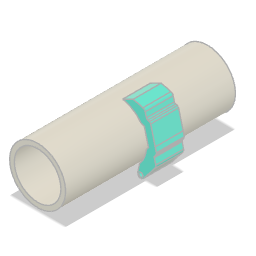
Payload Clamp Prototype (Autodesk Fusion 360 design; units mm, degrees)
Autodesk Fusion 360 part; units mm, degrees
sketch "Sketch1" plane through (0, 0, 0) normal (0, 0, 1) x (1, 0, 0)
  circle A0 centre (0, 50) radius 30
  circle A1 centre (0, 50) radius 25
  dimension "d1" = 60
  dimension "d2" = -5
  measures "d1" diameter of A0
extrude "Extrude1" add sketch "Sketch1" along normal blind 175 makes body 1
extrude "Extrude2" add sketch "Sketch1" against normal blind 7.5 contours A0 | A1 bodies 1
sketch "Sketch2" plane through (0, 0, -7.5) normal (0, 0, -1) x (-1, 0, 0)
  circle A0 centre (0, 50) radius 30
  circle A1 centre (0, 50) radius 30
  line L0 (0, 20) -> (0, 25)
  line L1 (-18.3303, 25) -> (-16.5831, 25)
  line L2 (-23.608, 29.9087) -> (-34.5881, 29.9087)
  line L3 (-30.7813, 46.3244) -> (-39.3496, 42.8163)
  circle A2 centre (0, 50) radius 31
  line L4 (-24.7175, 68.7094) -> (-27.8021, 78.7583)
  line L5 (-5.2295, 80.5557) -> (-16.7866, 86.3071)
  arc A3 (-16.7866, 86.3071) -> (-27.8021, 78.7583) centre (0, 50) ccw
  arc A4 (-39.3496, 42.8163) -> (-34.5881, 29.9087) centre (0, 50) ccw
  line L6 (5.2295, 80.5557) -> (16.7866, 86.3071)
  arc A5 (27.8021, 78.7583) -> (16.7866, 86.3071) centre (0, 50) ccw
  line L7 (24.7175, 68.7094) -> (27.8021, 78.7583)
  line L8 (30.7813, 46.3244) -> (39.3496, 42.8163)
  arc A6 (34.5881, 29.9087) -> (39.3496, 42.8163) centre (0, 50) ccw
  line L9 (23.608, 29.9087) -> (34.5881, 29.9087)
  dimension "d8" = 1
  constraint coincident A0 L0.start
  constraint concentric A0 A3
  constraint coincident L2.end A3
  constraint horizontal L2
  constraint coincident L3.end A3
  constraint coincident A2 L3.start
  constraint coincident A2 L2.start
  constraint coincident A2 L4.start
  constraint coincident A2 L5.start
  constraint concentric A3 A4
  constraint coincident A0 L1.end
  constraint coincident A2 L1.start
  constraint symmetric L0 L2.end A6.start
  constraint symmetric L0 L3.end L8.end
  constraint symmetric L0 L3.start L8.start
  constraint symmetric L0 L2.start L9.start
  constraint symmetric L0 L4.start L7.start
  constraint symmetric L0 L4.end A5.start
  constraint symmetric L0 L5.start L6.start
  constraint symmetric L0 L5.end L6.end
  constraint symmetric L0 A3 A5
  constraint symmetric L0 A4 A6
extrude "Extrude3" add sketch "Sketch2" against normal blind 30 separate body contours L2 L3 A2 A4 | A2 L4 L5 A3 | A2 L8 A6 L9 | A2 L6 A5 L7 makes body 2 at (-7.7659, 80.0115, 12.5) makes body 3 at (30.5651, 44.8256, 2.5) makes body 4 at (23.9131, 69.7273, 12.5) makes body 5 at (-29.4818, 40.4174, 12.5)
sketch "Sketch3" plane through (0, 0, -7.5) normal (0, 0, -1) x (-1, 0, 0)
  line L0 (-5.2295, 80.5557) -> (-16.7866, 86.3071)
  arc A0 (-16.7866, 86.3071) -> (-27.8021, 78.7583) centre (0, 50) ccw
  line L1 (-27.8021, 78.7583) -> (-24.7175, 68.7094)
  arc A1 (-5.2295, 80.5557) -> (-24.7175, 68.7094) centre (0, 50) ccw
  line L2 (-30.7813, 46.3244) -> (-39.3496, 42.8163)
  arc A2 (-39.3496, 42.8163) -> (-34.5881, 29.9087) centre (0, 50) ccw
  line L3 (-34.5881, 29.9087) -> (-23.608, 29.9087)
  arc A3 (-30.7813, 46.3244) -> (-23.608, 29.9087) centre (0, 50) ccw
  circle A4 centre (0, 50) radius 30
  circle A5 centre (-37.528, 36.1563) radius 2.5
  arc A6 (-40.9187, 37.0242) -> (-39.5025, 33.2664) centre (-37.528, 36.1563) ccw
  circle A7 centre (-26.2598, 80.1732) radius 2.5
  arc A8 (-27.1572, 83.5562) -> (-29.6505, 81.0412) centre (-26.2598, 80.1732) ccw
  line L4 (-40.9187, 37.0242) -> (-29.6505, 81.0412)
  line L5 (-31.0003, 57.936) -> (-28.6395, 67.1583)
  line L6 (-31.0003, 57.936) -> (-33.1425, 49.5681)
  line L7 (-27.1572, 83.5562) -> (-16.7866, 86.3071)
  line L8 (-39.5025, 33.2664) -> (-34.5881, 29.9087)
  line L9 (-25.7516, 72.078) -> (-24.7175, 68.7094)
  line L10 (-33.1425, 49.5681) -> (-30.7813, 46.3244)
  line L11 (-24.7175, 68.7094) -> (-28.6395, 67.1583)
  dimension "d11" = 5
  dimension "d12" = 7
  dimension "d13" = 5
  dimension "d14" = 7
  constraint midpoint A2 A5.centre
  constraint concentric A5 A6
  constraint coincident A0 A7.centre
  constraint concentric A7 A8
  constraint tangent A6 L4
  constraint coincident A8 L4.end
  constraint tangent A8 L4
  constraint tangent A8 L7
  constraint coincident L0.end A0.start
  constraint tangent A6 L8
  constraint coincident A2.end L3.start
  constraint coincident L4 A8.end
  constraint coincident L1 L9.start
  constraint coincident L1.end A1.end
  constraint coincident L2.start A3.start
  measures "d11" diameter of A5
  measures "d12" diameter of A6
  measures "d13" diameter of A7
  measures "d14" diameter of A8
extrude "Extrude4" add sketch "Sketch3" against normal blind 30 contours A0 L1 L2 A2 A5 A6 A7 A8 L4 L5 L6 L7 L8 L9 L10 L11 bodies 3 4
extrude "Extrude5" cut sketch "Sketch3" against normal blind 30 contours A0 L1 A7 | A2 A5 picked at (-25.5221, 79.7151) picked at (-36.7243, 36.3975) bodies 3
delete_body "RemoveBody1" bodies 5
delete_body "RemoveBody2" bodies 2
copy_body "CopyPasteBodies1" bodies 3 makes body 6
move_body "Move1" bodies 6 to x (0.707107, -0.707107, 0) y (0.707107, 0.707107, 0) z (0, 0, 1) at (-7.5036, 30.0552, 0)
sketch "Sketch4" plane through (0, 0, -7.5) normal (0, 0, -1) x (-1, 0, 0)
  circle A0 centre (0, 50) radius 30
  circle A1 centre (-37.528, 36.1563) radius 2.5
  circle A2 centre (-44.5991, 29.0852) radius 2.5
  circle A3 centre (-24.8785, 20.0964) radius 2.5
  line L0 (-34.7785, 38.3219) -> (-22.1289, 22.2621)
  line L1 (-40.2775, 33.9906) -> (-27.628, 17.9307)
  arc A4 (-34.7785, 38.3219) -> (-40.2775, 33.9906) centre (-37.528, 36.1563) ccw
  arc A5 (-27.628, 17.9307) -> (-22.1289, 22.2621) centre (-24.8785, 20.0964) ccw
  dimension "d20" = 5
  dimension "d21" = 7
  dimension "d22" = 7
  constraint concentric A3 A5
  constraint concentric A1 A4
  constraint tangent L0 A4
  constraint tangent L0 A5
  constraint tangent L1 A4
  constraint tangent L1 A5
  constraint parallel L0 L1
  measures "d20" diameter of A3
  measures "d21" diameter of A5
  measures "d22" diameter of A4
extrude "Extrude6" add sketch "Sketch4" along normal blind 7.5 separate body contours L0 L1 A4 A5 makes body 7
move_body "Move2" bodies 7 to x (0.906308, -0.422618, 0) y (0.422618, 0.906308, 0) z (0, 0, 1) at (-6.1622, 12.397, 0)
move_body "Move3" bodies 6 to x (1, 0, 0) y (0, 1, 0) z (0, 0, 1) at (-1.5, 0.25, 0)
move_body "Move4" bodies 7 to x (0.906308, 0.422618, 0) y (-0.422618, 0.906308, 0) z (0, 0, 1) at (10.824, -8.6312, 0)
sketch "Sketch5" plane through (0, 0, -7.5) normal (0, 0, -1) x (-1, 0, 0)
  circle A0 centre (-26.2598, 80.1732) radius 2.5
  line L0 (-34.5881, 29.9087) -> (-23.608, 29.9087)
  arc A1 (-30.7813, 46.3244) -> (-23.608, 29.9087) centre (0, 50) ccw
  line L1 (-30.7813, 46.3244) -> (-33.1425, 49.5681)
  line L2 (-33.1425, 49.5681) -> (-28.6395, 67.1583)
  line L3 (-28.6395, 67.1583) -> (-24.7175, 68.7094)
  arc A2 (-5.2295, 80.5557) -> (-24.7175, 68.7094) centre (0, 50) ccw
  line L4 (-5.2295, 80.5557) -> (-16.7866, 86.3071)
  line L5 (-16.7866, 86.3071) -> (-27.1572, 83.5562)
  arc A3 (-27.1572, 83.5562) -> (-29.6505, 81.0412) centre (-26.2598, 80.1732) ccw
  line L6 (-29.6505, 81.0412) -> (-40.9187, 37.0242)
  arc A4 (-40.9187, 37.0242) -> (-39.5025, 33.2664) centre (-37.528, 36.1563) ccw
  line L7 (-39.5025, 33.2664) -> (-34.5881, 29.9087)
  circle A5 centre (-37.528, 36.1563) radius 2.5
  circle A6 centre (-26.2598, 80.1732) radius 2.5
  line L8 (-58.0759, 36.6699) -> (-29.6505, 81.0412)
  line L9 (-23.3075, 78.2934) -> (-49.9806, 36.4014)
  circle A7 centre (-24.8785, 20.0964) radius 2.5
  line L10 (-56.5521, 31.863) -> (-26.4306, 16.9594)
  line L11 (-23.3282, 23.2344) -> (-49.9806, 36.4014)
  arc A8 (-23.3075, 78.2934) -> (-29.6505, 81.0412) centre (-26.2598, 80.1732) ccw
  arc A9 (-26.4306, 16.9594) -> (-23.3282, 23.2344) centre (-24.8785, 20.0964) ccw
  arc A10 (-57.8029, 37.0962) -> (-56.5521, 31.863) centre (-55, 35) ccw
  dimension "d25" = 7
  dimension "d26" = 7
  dimension "d27" = 7
  constraint concentric A6 A8
  constraint coincident L8.start A10
  constraint coincident A3.end L6.start
  constraint tangent L9 A8
  constraint concentric A7 A9
  constraint tangent L10 A10
  constraint tangent L10 A9
  constraint tangent L11 A9
  constraint coincident L8 A10.start
  measures "d25" diameter of A8
  measures "d26" diameter of A10
  measures "d27" diameter of A9
extrude "Extrude7" add sketch "Sketch5" along normal blind 7.5 separate body contours L6 L8 L9 L10 L11 A9 A10 | A3 L6 L9 A8 makes body 8
delete_body "RemoveBody3" bodies 8
move_body "Move5" bodies 7 to x (1, 0, 0) y (0, 1, 0) z (0, 0, 1) at (0, 0, 38)
extrude "Extrude8" add 1 faces at (35.3299, 28.5468, 30.5) along direction (0, 0, 1) blind 20 on bodies 7 bodies 7
sketch "Sketch6" plane through (0, 0, 23) normal (0, 0, -1) x (-1, 0, 0)
  circle A0 centre (-37.528, 36.1563) radius 2.5
  circle A1 centre (-24.8785, 20.0964) radius 2.5
  arc A2 (-34.7785, 38.3219) -> (-40.2775, 33.9906) centre (-37.528, 36.1563) ccw
  line L0 (-40.2775, 33.9906) -> (-27.628, 17.9307)
  arc A3 (-27.628, 17.9307) -> (-22.1289, 22.2621) centre (-24.8785, 20.0964) ccw
  line L1 (-22.1289, 22.2621) -> (-34.7785, 38.3219)
  circle A4 centre (-24.8785, 20.0964) radius 2.5
  line L2 (-21.4618, 15.0964) -> (-14.8785, 15.0964)
  line L3 (-14.8785, 15.0964) -> (-14.8785, 10.0964)
  line L4 (-14.8785, 10.0964) -> (-24.8785, 10.0964)
  line L5 (-28.3785, 15.0964) -> (-34.8785, 15.0964)
  line L6 (-34.8785, 15.0964) -> (-34.8785, 10.0964)
  line L7 (-34.8785, 10.0964) -> (-24.8785, 10.0964)
  line L8 (-21.3789, 20.0377) -> (-21.4618, 15.0964)
  line L9 (-28.3785, 20.0964) -> (-28.3785, 15.0964)
  arc A5 (-21.3789, 20.0377) -> (-28.3785, 20.0964) centre (-24.8785, 20.0964) ccw
  dimension "d32" = 7
  constraint concentric A4 A5
  constraint horizontal L2
  constraint vertical L3
  constraint horizontal L4
  constraint horizontal L5
  constraint vertical L6
  constraint horizontal L7
  constraint coincident A3 L8.start
  constraint tangent L8 A5
  constraint tangent L9 A5
  constraint perpendicular L5 L9
  measures "d32" diameter of A5
extrude "Extrude9" add sketch "Sketch6" along normal blind 8 separate body contours L0 A3 L9 A5 | L0 A3 L2 L3 L4 L5 L6 L7 L8 L9 makes body 9
fillet "Fillet1" radius 4 2 edges at (28.3785, 15.0964, 19) (21.4618, 15.0964, 19) on bodies 9
sketch "Sketch7" plane through (0, 0, 23) normal (0, 0, 1) x (1, 0, 0)
  circle A0 centre (24.8785, 20.0964) radius 2.5
  line L0 (21.3789, 20.0377) -> (21.3936, 19.1635)
  arc A1 (17.3942, 15.0964) -> (21.3936, 19.1635) centre (17.3942, 19.0964) ccw
  line L1 (17.3942, 15.0964) -> (14.8785, 15.0964)
  line L2 (14.8785, 15.0964) -> (14.8785, 10.0964)
  line L3 (14.8785, 10.0964) -> (34.8785, 10.0964)
  line L4 (34.8785, 10.0964) -> (34.8785, 15.0964)
  line L5 (34.8785, 15.0964) -> (32.3785, 15.0964)
  arc A2 (28.3785, 19.0964) -> (32.3785, 15.0964) centre (32.3785, 19.0964) ccw
  line L6 (28.3785, 19.0964) -> (28.3785, 20.0964)
  arc A3 (28.3785, 20.0964) -> (21.3789, 20.0377) centre (24.8785, 20.0964) ccw
  circle A4 centre (24.8785, 20.0964) radius 2.5
extrude "Extrude10" add sketch "Sketch7" along normal blind -8 and the other way blind -16 contours A0 A4 bodies 9
extrude "Extrude11" cut 1 faces at (25.6495, 19.2654, 39) along direction (0, 0, -1) blind 15 on bodies 9 bodies 9
sketch "Sketch8" plane through (0, 0, 24) normal (0, 0, 1) x (1, 0, 0)
  circle A0 centre (24.8785, 20.0964) radius 2.5
  circle A1 centre (24.8785, 20.0964) radius 2.3
  dimension "d47" = -0.2
extrude "Extrude12" add sketch "Sketch8" along normal blind 35 contours A1 bodies 9
extrude "Extrude13" cut 1 faces at (23.27, 18.2787, 24) along direction (0, 0, -1) blind 1 on bodies 9 bodies 9
extrude "Extrude14" cut 2 faces at (27.3025, 19.9722, 23) (23.1114, 11.9792, 23) along direction (0, 0, -1) blind 0.2 on bodies 9 bodies 9
copy_body "Body->Comp1" bodies 9 removing the originals makes body 10 in component "Body Hinge Mount"
copy_body "Body->Comp2" bodies 7 removing the originals makes body 11 in component "Lower Pivot"
sketch "Sketch9" plane through (0, 0, 23) normal (0, 0, -1) x (-1, 0, 0)
  circle A0 centre (-37.528, 36.1563) radius 2.5
  circle A1 centre (-24.8785, 20.0964) radius 2.5
  arc A2 (-34.7785, 38.3219) -> (-40.2775, 33.9906) centre (-37.528, 36.1563) ccw
  line L0 (-40.2775, 33.9906) -> (-27.628, 17.9307)
  arc A3 (-27.628, 17.9307) -> (-22.1289, 22.2621) centre (-24.8785, 20.0964) ccw
  line L1 (-22.1289, 22.2621) -> (-34.7785, 38.3219)
  circle A4 centre (-37.528, 36.1563) radius 2.5
extrude "Extrude1'" add sketch "Sketch9" against normal blind 28 contours A0 A4 bodies 11 in component "Lower Pivot"
sketch "Sketch10" plane through (0, 0, 23) normal (0, 0, -1) x (-1, 0, 0)
  circle A0 centre (-24.8785, 20.0964) radius 2.5
  arc A1 (-34.7785, 38.3219) -> (-40.2775, 33.9906) centre (-37.528, 36.1563) ccw
  line L0 (-40.2775, 33.9906) -> (-27.628, 17.9307)
  arc A2 (-27.628, 17.9307) -> (-22.1289, 22.2621) centre (-24.8785, 20.0964) ccw
  line L1 (-22.1289, 22.2621) -> (-34.7785, 38.3219)
  circle A3 centre (-37.528, 36.1563) radius 2.5
  circle A4 centre (-37.528, 36.1563) radius 2.3
  dimension "d63" = -0.2
extrude "Extrude2'" add sketch "Sketch10" along normal blind 4 contours A4 bodies 11 in component "Lower Pivot"
extrude "Extrude3'" cut 1 faces at (36.8049, 36.3964, 51) along direction (0, 0, -1) blind 0.5 on bodies 11 bodies 11 in component "Lower Pivot"
extrude "Extrude4'" add 1 faces at (36.7954, 35.9303, 19) along direction (0, 0, -1) blind 30 on bodies 11 bodies 11 in component "Lower Pivot"
copy_body "Body->Comp3" bodies 3 removing the originals makes body 12 in component "clamp"
delete_body "RemoveBody7" bodies 6
delete_face "DeleteFace1" 1 faces at (24.0487, 81.3397, 12.5) on bodies 12 in component "clamp"
extrude "Extrude5'" cut 1 faces at (36.7954, 35.9303, -11) along direction (0, 0, 1) blind 34 on bodies 11 bodies 11 in component "Lower Pivot"
delete_face "DeleteFace2" 1 faces at (38.5517, 38.4371, 2.5) on bodies 12 in component "clamp"
sketch "Sketch11" plane through (0, 0, 59) normal (0, 0, -1) x (-1, 0, 0)
  line L0 (-34.5881, 29.9087) -> (-23.608, 29.9087)
  arc A0 (-30.7813, 46.3244) -> (-23.608, 29.9087) centre (0, 50) ccw
  line L1 (-30.7813, 46.3244) -> (-33.1425, 49.5681)
  line L2 (-33.1425, 49.5681) -> (-28.6395, 67.1583)
  line L3 (-28.6395, 67.1583) -> (-24.7175, 68.7094)
  arc A1 (-5.2295, 80.5557) -> (-24.7175, 68.7094) centre (0, 50) ccw
  line L4 (-5.2295, 80.5557) -> (-16.7866, 86.3071)
  line L5 (-16.7866, 86.3071) -> (-27.1572, 83.5562)
  arc A2 (-27.1572, 83.5562) -> (-29.6505, 81.0412) centre (-26.2598, 80.1732) ccw
  line L6 (-29.6505, 81.0412) -> (-40.9187, 37.0242)
  arc A3 (-40.9187, 37.0242) -> (-39.5025, 33.2664) centre (-37.528, 36.1563) ccw
  line L7 (-39.5025, 33.2664) -> (-34.5881, 29.9087)
  circle A4 centre (-24.8785, 20.0964) radius 2.3
  circle A5 centre (-24.8785, 20.0964) radius 3.5
  line L8 (-21.4729, 20.9039) -> (-23.608, 29.9087)
  line L9 (-27.628, 17.9307) -> (-40.2775, 33.9906)
  dimension "d78" = 7
  constraint concentric A4 A5
  constraint coincident A5 L8.start
  constraint tangent A5 L8
  constraint coincident L0.end A0.end
  constraint coincident A5 L9.start
  constraint tangent A5 L9
  constraint coincident A3 L9.end
  constraint tangent A3 L9
  measures "d78" diameter of A5
extrude "Extrude1''" add sketch "Sketch11" against normal blind 30 contours L0 A3 L7 A5 L8 L9 | A5 sketch seen with x (1, 0, 0) y (0, 1, 0) z (0, 0, 1) at (0, 0, -66.5) bodies 12 in component "clamp"
sketch "Sketch12" plane through (0, 0, 59) normal (0, 0, -1) x (-1, 0, 0)
  circle A0 centre (-24.8785, 20.0964) radius 2.3
  arc A1 (-30.7813, 46.3244) -> (-23.608, 29.9087) centre (0, 50) ccw
  line L0 (-30.7813, 46.3244) -> (-33.1425, 49.5681)
  line L1 (-33.1425, 49.5681) -> (-28.6395, 67.1583)
  line L2 (-28.6395, 67.1583) -> (-24.7175, 68.7094)
  arc A2 (-5.2295, 80.5557) -> (-24.7175, 68.7094) centre (0, 50) ccw
  line L3 (-5.2295, 80.5557) -> (-16.7866, 86.3071)
  line L4 (-16.7866, 86.3071) -> (-27.1572, 83.5562)
  arc A3 (-27.1572, 83.5562) -> (-29.6505, 81.0412) centre (-26.2598, 80.1732) ccw
  line L5 (-29.6505, 81.0412) -> (-40.9187, 37.0242)
  arc A4 (-40.9187, 37.0242) -> (-40.2775, 33.9906) centre (-37.528, 36.1563) ccw
  line L6 (-40.2775, 33.9906) -> (-27.628, 17.9307)
  arc A5 (-27.628, 17.9307) -> (-21.4729, 20.9039) centre (-24.8785, 20.0964) ccw
  line L7 (-21.4729, 20.9039) -> (-23.608, 29.9087)
  line L8 (-28.8485, 66.3417) -> (-36.5986, 68.3257)
  line L9 (-32.5853, 51.7447) -> (-40.3354, 53.7287)
  line L10 (-40.3354, 53.7287) -> (-36.5986, 68.3257)
  line L11 (-31.9619, 47.9463) -> (-38.4298, 43.2382)
  line L12 (-38.4298, 43.2382) -> (-41.8568, 47.9463)
  line L13 (-41.8568, 47.9463) -> (-40.3354, 53.7287)
  line L14 (-26.6785, 67.9339) -> (-28.9259, 75.6117)
  line L15 (-28.9259, 75.6117) -> (-35.2038, 73.7741)
  line L16 (-35.2038, 73.7741) -> (-36.5986, 68.3257)
  dimension "d81" = 8
  dimension "d82" = 8
  dimension "d83" = 8
  dimension "d84" = 8
  constraint coincident L1 L8.start
  constraint perpendicular L1 L8
  constraint coincident L1 L9.start
  constraint perpendicular L1 L9
  constraint perpendicular L8 L10
  constraint midpoint L0 L11.start
  constraint perpendicular L0 L11
  constraint perpendicular L11 L12
  constraint midpoint L2 L14.start
  constraint perpendicular L14 L15
  constraint perpendicular L8 L16
  measures "d81" distance of L8.start L8.end
  measures "d82" distance of L9.start L9.end
  measures "d83" distance of L11.start L11.end
  measures "d84" distance of L14.start L14.end
extrude "Extrude2''" add sketch "Sketch12" against normal blind 30 contours L5 L9 L12 L13 | L5 L8 L9 L10 | L5 L8 L15 L16 sketch seen with x (1, 0, 0) y (0, 1, 0) z (0, 0, 1) at (0, 0, -66.5) bodies 12 in component "clamp"
fillet "Fillet1'" radius 2 4 edges at (31.2117, 74.9426, 7.5) (35.2038, 73.7741, 7.5) (39.0942, 44.151, 7.5) (41.8568, 47.9463, 7.5) on bodies 12 in component "clamp"
component "Body Hinge Mount" placed x (1, 0, 0) y (0, 1, 0) z (0, 0, 1) at (0, 0, 0)
component "Lower Pivot" placed x (1, 0, 0) y (0, 1, 0) z (0, 0, 1) at (0, 0, 0)
component "clamp" placed x (1, 0, 0) y (0, 1, 0) z (0, 0, 1) at (0, 0, -0.5)
component "Body Hinge Mount" placed x (1, 0, 0) y (0, 1, 0) z (0, 0, 1) at (0, 0, 67)
component "Lower Pivot" placed x (1, 0, 0) y (0, 1, 0) z (0, 0, 1) at (0, 0, 67)
component "clamp" placed x (1, 0, 0) y (0, 1, 0) z (0, 0, 1) at (0, 0, 66.5)
named bodies: "cyl", "clamp", "clamp (1)", "Lower Pivot", "Body Hinge Mount"
